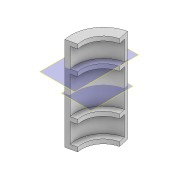
# Autodesk Inventor part: circular_tether
Saved by Autodesk Inventor 2021 (Build 250183000, 183)
## iProperties
Created: 2021-03-03
Part Number: circular_tether
Material: Generic
Document SubType Name: Modeling
Designer: Sihan
Density: 1 g/cm^3
Appearance: Default
Mass: 0.296755 g
Surface Area: 6.62196 cm^2
Volume: 0.296755 cm^3
Author: Sihan
Autodesk Inventor part; units mm, degrees
ref_plane "YZ Plane" through (0, 0, 0) normal (1, 0, 0) x (0, 1, 0)
ref_plane "XZ Plane" through (0, 0, 0) normal (0, 1, 0) x (-1, 0, 0)
ref_plane "XY Plane" through (0, 0, 0) normal (0, 0, 1) x (1, 0, 0)
sketch "Sketch1" plane through (0, 0, 0) normal (0, 1, 0) x (-1, 0, 0)
  arc A0 (1.6544, -7.3153) -> (7.3153, 1.6544) centre (0, 0) ccw
  arc A1 (1.4338, -6.3399) -> (6.3399, 1.4338) centre (0, 0) ccw
  line L0 (7.3153, 1.6544) -> (6.3399, 1.4338)
  line L1 (1.4338, -6.3399) -> (1.6544, -7.3153)
  dimension "d0" = 7.5
  dimension "d1" = 1
  dimension "d4" = 90
  constraints: 4 end point, 4 point on circle, 2 centre point, 1 coincident
  measures "d0" radius of A0
  measures "d1" radial gap between concentric circles of A0 A1
extrude "Extrusion1" add sketch "Sketch1" along normal mid plane 19.821
sketch "Sketch2" plane through (0, 9.9105, 0) normal (0, 1, 0) x (1, 0, 0)
  arc A0 (-1.6544, 7.3153) -> (-7.3153, -1.6544) centre (0, 0) ccw projected
  arc A1 (-1.1029, 4.8768) -> (-4.8768, -1.1029) centre (0, 0) ccw
  line L0 (-7.3153, -1.6544) -> (-4.8768, -1.1029)
  line L1 (-1.1029, 4.8768) -> (-1.6544, 7.3153)
  line L2 (-7.3153, -1.6544) -> (-6.3399, -1.4338) projected
  line L3 (-1.4338, 6.3399) -> (-1.6544, 7.3153) projected
  dimension "d9" = 2.5
  constraints: 4 end point, 3 point on circle, 2 collinear, 1 centre point
  measures "d9" radial gap between concentric circles of A0 A1
extrude "Extrusion2" add sketch "Sketch2" along normal blind 1
mirror "Mirror1" about plane through (0, 0, 0) normal (0, 1, 0) of "Extrusion2"
ref_plane "Work Plane2" through (0, 5.3105, 0) normal (0, -1, 0) x (1, 0, 0)
sketch "Sketch3" plane through (0, 5.3105, 0) normal (0, -1, 0) x (1, 0, 0)
  arc A0 (-7.3153, 1.6544) -> (-1.6544, -7.3153) centre (0, 0) ccw projected
  line L0 (-7.3153, 1.6544) -> (-4.8768, 1.1029) projected
  arc A1 (-4.8768, 1.1029) -> (-1.1029, -4.8768) centre (0, 0) ccw projected
  line L1 (-1.1029, -4.8768) -> (-1.6544, -7.3153) projected
extrude "Extrusion3" add sketch "Sketch3" along normal blind 1
mirror "Mirror2" about plane through (0, 0, 0) normal (0, 1, 0) of "Extrusion3"
ref_plane "Work Plane3" through (-6.3399, 12.512, 1.4338) normal (-0.8457, 0, -0.5337) x (0.5337, 0, -0.8457)
sketch "Sketch4" plane through (-14.3948, 12.512, -3.6499) normal (-0.8457, 0, -0.5337) x (0.5337, 0, -0.8457)
  line L0 (3.7075, 16.0789) -> (7.5195, 16.0789) construction
  line L1 (7.5195, 16.0789) -> (7.5195, 13.4854) construction
  line L2 (7.5195, 13.4854) -> (3.7075, 13.4854) construction
  line L3 (3.7075, 13.4854) -> (3.7075, 16.0789) construction
  point P0 (4.5962, 12.512)
  constraints: 2 other
ref_plane "Work Plane1" through (0, 0, 0) normal (0, 1, 0) x (-1, 0, 0)
body "Solid1"
body "Srf1"
body "Solid2"
body "Solid3"
